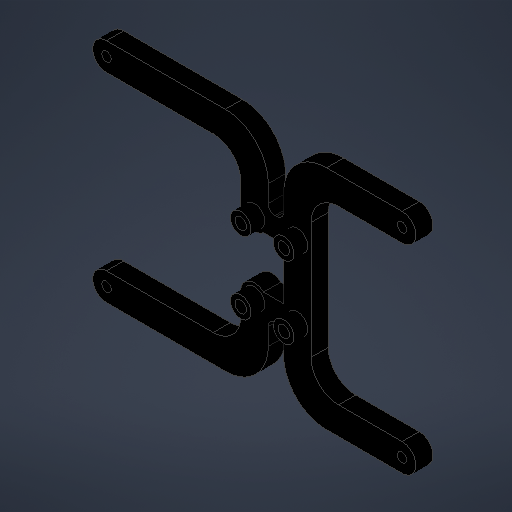
# Autodesk Inventor part: Camera Bracket
Saved by Autodesk Inventor 2026.1 (Build 301233020, 233B)
## iProperties
Created: 2025-12-28
Part Number: Camera Bracket
Material: Generic
Document SubType Name: Modeling
Designer: Bahaa
Density: 1 g/cm^3
Appearance: Default
Author: Bahaa
Autodesk Inventor part; units mm, degrees
ref_plane "YZ Plane" through (0, 0, 0) normal (1, 0, 0) x (0, 1, 0)
ref_plane "XZ Plane" through (0, 0, 0) normal (0, 1, 0) x (-1, 0, 0)
ref_plane "XY Plane" through (0, 0, 0) normal (0, 0, 1) x (1, 0, 0)
sketch "Sketch1" plane through (0, 0, 0) normal (0, 1, 0) x (-1, 0, 0)
  line L0 (0, 0) -> (9.45, 0) construction
  line L1 (0, 0) -> (-14.55, 0) construction
  line L2 (9.45, 0) -> (-14.55, 0) construction
  line L3 (-14.55, 12.5) -> (9.45, 12.5) construction
  line L4 (9.45, 12.5) -> (9.45, -12.5) construction
  line L5 (9.45, -12.5) -> (-14.55, -12.5) construction
  line L6 (-14.55, -12.5) -> (-14.55, 12.5) construction
  line L7 (-14.55, 12.5) -> (9.45, -12.5) construction
  line L8 (9.45, 12.5) -> (-14.55, -12.5) construction
  line L9 (0, 10.5) -> (-12.5, 10.5) construction
  line L10 (0, 10.5) -> (0, 29) construction
  line L11 (0, 29) -> (43.05, 29) construction
  line L12 (-12.5, 10.5) -> (-12.5, 29) construction
  line L13 (-12.5, 29) -> (-42.95, 29) construction
  line L14 (43.05, 29) -> (0, 29) construction
  line L15 (43.05, 33) -> (0, 33)
  line L16 (0, 25) -> (43.05, 25)
  arc A0 (43.05, 25) -> (43.05, 33) centre (43.05, 29) ccw
  arc A1 (0, 33) -> (0, 25) centre (0, 29) ccw
  line L17 (0, 29) -> (0, 10.5) construction
  line L18 (-4, 29) -> (-4, 10.5)
  line L19 (4, 10.5) -> (4, 29)
  arc A2 (4, 29) -> (-4, 29) centre (0, 29) ccw
  arc A3 (-4, 10.5) -> (4, 10.5) centre (0, 10.5) ccw
  line L20 (-42.95, 29) -> (-12.5, 29) construction
  line L21 (-42.95, 25) -> (-12.5, 25)
  line L22 (-12.5, 33) -> (-42.95, 33)
  arc A4 (-42.95, 33) -> (-42.95, 25) centre (-42.95, 29) ccw
  arc A5 (-12.5, 25) -> (-12.5, 33) centre (-12.5, 29) ccw
  line L23 (-12.5, 29) -> (-12.5, 10.5) construction
  line L24 (-16.5, 29) -> (-16.5, 10.5)
  line L25 (-8.5, 10.5) -> (-8.5, 29)
  arc A6 (-8.5, 29) -> (-16.5, 29) centre (-12.5, 29) ccw
  arc A7 (-16.5, 10.5) -> (-8.5, 10.5) centre (-12.5, 10.5) ccw
  line L26 (0, 10.5) -> (-12.5, 10.5) construction
  line L27 (0, 13.5) -> (-12.5, 13.5)
  line L28 (-12.5, 7.5) -> (0, 7.5)
  arc A8 (0, 7.5) -> (0, 13.5) centre (0, 10.5) ccw
  arc A9 (-12.5, 13.5) -> (-12.5, 7.5) centre (-12.5, 10.5) ccw
  circle A10 centre (0, 10.5) radius 3
  circle A11 centre (-12.5, 10.5) radius 3
  line L29 (-16.5, 10.5) -> (-16.5, -1.75)
  line L30 (-4, 33) -> (4, 33)
  line L31 (4, 33) -> (4, 25)
  line L32 (4, 25) -> (-4, 25)
  line L33 (-4, 25) -> (-4, 33)
  line L34 (-4, 33) -> (4, 25) construction
  line L35 (4, 33) -> (-4, 25) construction
  line L36 (-8.5, 33) -> (-16.5, 33)
  line L37 (-16.5, 33) -> (-16.5, 25)
  line L38 (-16.5, 25) -> (-8.5, 25)
  line L39 (-8.5, 25) -> (-8.5, 33)
  line L40 (-8.5, 33) -> (-16.5, 25) construction
  line L41 (-16.5, 33) -> (-8.5, 25) construction
  line L42 (0, -10.5) -> (0, -29) construction
  line L43 (0, -29) -> (43.05, -29) construction
  line L44 (-12.5, -10.5) -> (-12.5, -29) construction
  line L45 (-12.5, -29) -> (-42.95, -29) construction
  line L46 (43.05, -29) -> (0, -29) construction
  line L47 (43.05, -33) -> (0, -33)
  line L48 (0, -25) -> (43.05, -25)
  arc A12 (43.05, -33) -> (43.05, -25) centre (43.05, -29) ccw
  arc A13 (0, -25) -> (0, -33) centre (0, -29) ccw
  line L49 (0, -29) -> (0, -10.5) construction
  line L50 (-4, -29) -> (-4, -10.5)
  line L51 (4, -10.5) -> (4, -29)
  arc A14 (-4, -29) -> (4, -29) centre (0, -29) ccw
  line L52 (-42.95, -29) -> (-12.5, -29) construction
  line L53 (-42.95, -25) -> (-12.5, -25)
  line L54 (-12.5, -33) -> (-42.95, -33)
  arc A15 (-42.95, -25) -> (-42.95, -33) centre (-42.95, -29) ccw
  arc A16 (-12.5, -33) -> (-12.5, -25) centre (-12.5, -29) ccw
  line L55 (-12.5, -29) -> (-12.5, -10.5) construction
  line L56 (-16.5, -29) -> (-16.5, -10.5)
  line L57 (-8.5, -10.5) -> (-8.5, -29)
  arc A17 (-16.5, -29) -> (-8.5, -29) centre (-12.5, -29) ccw
  line L58 (0, -10.5) -> (-12.5, -10.5) construction
  line L59 (0, -13.5) -> (-12.5, -13.5)
  line L60 (-12.5, -7.5) -> (0, -7.5)
  arc A18 (-12.5, -7.5) -> (-12.5, -13.5) centre (-12.5, -10.5) ccw
  circle A19 centre (0, -10.5) radius 3
  circle A20 centre (-12.5, -10.5) radius 3
  line L61 (-16.5, -10.5) -> (-16.5, -1.75)
  line L62 (-4, -33) -> (4, -33)
  line L63 (4, -33) -> (4, -25)
  line L64 (4, -25) -> (-4, -25)
  line L65 (-4, -25) -> (-4, -33)
  line L66 (-4, -33) -> (4, -25) construction
  line L67 (4, -33) -> (-4, -25) construction
  line L68 (-8.5, -33) -> (-16.5, -33)
  line L69 (-16.5, -33) -> (-16.5, -25)
  line L70 (-16.5, -25) -> (-8.5, -25)
  line L71 (-8.5, -25) -> (-8.5, -33)
  line L72 (-8.5, -33) -> (-16.5, -25) construction
  line L73 (-16.5, -33) -> (-8.5, -25) construction
  circle A21 centre (-42.95, 29) radius 1.35
  circle A22 centre (-42.95, -29) radius 1.35
  circle A23 centre (43.05, 29) radius 1.35
  circle A24 centre (43.05, -29) radius 1.35
  line L74 (-8.5, 10.5) -> (-8.5, -10.5)
  circle A25 centre (0, -10.5) radius 4
  line L75 (-6.25, 10.5) -> (-6.25, -10.5) construction
  point P0 (-2.55, 0)
  point P1 (21.525, 29)
  point P2 (0, 19.75)
  point P3 (-27.725, 29)
  point P4 (-12.5, 19.75)
  point P5 (21.525, -29)
  point P6 (-27.725, -29)
  point P7 (-8.5, -13.5)
  point P8 (-4, -13.5)
  point P9 (-4, -25)
  point P10 (4, -33)
  point P11 (4, -10.5)
  point P12 (0, -7.5)
  point P13 (-2.6458, 7.5)
  point P14 (0, 33)
  point P15 (-4, 29)
  point P16 (-4, 13.5)
  point P17 (-8.5, 13.5)
  point P18 (-12.5, -7.5)
  point P19 (-4, 10.5)
  point P20 (4, 10.5)
  point P21 (-8.5, 10.5)
  point P22 (4, -33)
  point P23 (-8.5, -7.5)
  point P24 (-8.5, 7.5)
  point P25 (-9.8542, 7.5)
  point P26 (-8.5, -29)
  point P27 (-12.5, -33)
  point P28 (-16.5, -29)
  point P29 (-12.5, -33)
  point P30 (4, 33)
  point P31 (-4, -29)
  point P32 (0, -33)
  point P33 (-4, -29)
  point P34 (-4, -10.5)
  point P35 (0, -33)
  point P36 (-8.5, -29)
  point P37 (-12.5, -33)
  point P38 (0, -33)
  point P39 (-8.5, 29)
  point P40 (-12.5, 33)
  point P41 (-12.5, 33)
  point P42 (-12.5, 33)
  point P43 (-12.5, 6.5)
  point P44 (0, 33)
  point P45 (-8.5, 29)
  point P46 (-4, 29)
  point P47 (0, 33)
  point P48 (4, 10.5)
  point P49 (0, 33)
  point P50 (0, 6.5)
  point P51 (0, -33)
  point P52 (-4, 10.5)
  point P53 (4, 10.5)
  point P54 (-12.5, 7.5)
  point P55 (-8.5, 10.5)
  point P56 (-12.5, 7.5)
  point P57 (0, 33)
  point P58 (-2.6458, -7.5)
  point P59 (0, 7.5)
  point P60 (-12.5, -25)
  dimension "d0" = 9.45
  dimension "d1" = 14.55
  dimension "d2" = 24
  dimension "d3" = 25
  dimension "d4" = 2
  dimension "d5" = 9.45
  dimension "d8" = 12.5
  dimension "d9" = 18.5
  dimension "d10" = 43.05
  dimension "d11" = 30.45
  dimension "d12" = 18.5
  dimension "d13" = 8
  dimension "d14" = 4
  dimension "d15" = 4
  dimension "d16" = 4
  dimension "d17" = 3
  dimension "d23" = 2.7
  dimension "d24" = 2.7
  dimension "d25" = 2.7
  dimension "d26" = 2.7
  constraints: 172 end point, 38 symmetric about line, 34 point on circle, 22 centre point, 21 tangent, 13 midpoint, 12 parallel, 11 coincident, 10 horizontal, 8 point on line, 4 collinear, 4 perpendicular, 4 vertical, 19 other
  measures "d0" distance of L0.start L0.end
  measures "d1" distance of L0.start L1.end
  measures "d2" distance of L4.end L5.end
  measures "d3" distance of L3.end L4.end
  measures "d4" distance from line of L3 L9.start
  measures "d5" distance from line of L4 L9.start
  measures "d8" distance of L9.start L9.end
  measures "d9" distance of L9.start L10.end
  measures "d10" distance of L10.end L11.end
  measures "d11" distance of L12.end L13.end
  measures "d12" distance of L12.start L12.end
  measures "d13" diameter of A1
  measures "d14" radius of A2
  measures "d15" radius of A5
  measures "d16" radius of A6
  measures "d17" radius of A8
  measures "d23" diameter of A21
  measures "d24" diameter of A22
  measures "d25" diameter of A23
  measures "d26" diameter of A24
extrude "Extrusion1" add sketch "Sketch1" along normal blind 5
extrude "Extrusion2" add sketch "Sketch1" against normal blind 4 contours A10 A8 | A11 A9 | A20 A18 | A19
fillet "Fillet1" radius 8 4 edges at (16.5, 2.5, 25) (16.5, 2.5, -25) (-4, 2.5, -25) (-4, 2.5, 25)
fillet "Fillet2" radius 12.5 4 edges at (4, 2.5, 33) (8.5, 2.5, 33) (8.5, 2.5, -33) (4, 2.5, -33)
fillet "Fillet3" radius 2 4 edges at (4, 2.5, 13.5) (8.5, 2.5, 13.5) (4, 2.5, -13.5) (8.5, 2.5, 7.5)
sketch "Sketch3" plane through (0, -4, 10.5) normal (0, -1, 0) x (1, 0, 0)
  arc A0 (-4, 0) -> (2.6458, -3) centre (0, 0) ccw projected
  circle A1 centre (12.5, 0) radius 3 projected
  circle A2 centre (12.5, -21) radius 3 projected
  circle A3 centre (0, -21) radius 3 projected
  point P0 (0, -10.5)
  point P1 (12.5, -3)
  point P2 (12.5, -24)
  point P3 (0, -18)
  point P4 (-4, -21)
  point P5 (0, -24)
  constraints: 4 coincident, 2 vertical alignment
hole "Hole2" at (0, -4, 10.5) at (12.5, -4, 10.5) at (12.5, -4, -10.5) at (0, -4, -10.5) direction (0, 1, 0) diameter 3.3 depth 4
equation "\"d5\" = d0"
equation "\"d12\" = d9"
body "Solid1"
